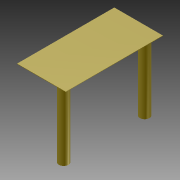
# Autodesk Inventor part: A11P-toggle-terminals
Saved by Autodesk Inventor 2011 SP1 (Build 150282100, 282)
## iProperties
Created: 2013-12-24
Part Number: A11P-toggle-terminals
Catalog Web Link: www.cadenas.de
Description: A Series - Process Sealed Subminiature Toggle - terminals-
Vendor: NKKSWITCHES
Document SubType Name: Modeling
Designer: PARTuser1
Manufacturer: NKKSWITCHES
Density: 1 g/cm^3
Category: PARTsolutions
Company: NKKSWITCHES
Title: A11P-toggle-terminals
Author: Cadenas PARTsolutions
PSOL_IDENT_0: {$CADENAS_DATA\23d-libs\nkkswitches\toggle\a\parts\a_toggle_terminals.prj},251 {VTYP=3D},{NB=A11P-to
PSOL_IDENT_1: ggle-terminals},{LINA=A11P-toggle-terminals},{NN=A Series - Process Sealed Subminiature Toggle - ter
PSOL_IDENT_2: minals},{DATE=05.03.2009 11:13:08},{GEOMDATE=05.03.2009 00:00:00},{VERSION=},{LINEID=10},{LINESUBID=
PSOL_IDENT_3: -1},{WBVAR=PLS,TRMNLS,CRCTS}  {NB=A11P-toggle-terminals},{LINA=A11P-toggle-terminals},{KT=DUMMY},{PN
PSOL_IDENT_4: =A11P},{SRS=A},{PLS=1},{TRMNLS=P},{TRMNLS1= 'P', 'P - Straight', 'B', 'B - Straight with Bracket', '
PSOL_IDENT_5: B1', 'B1 - Straight with Inline Bracket', 'H', 'H - Right Angle with Bracket', 'V', 'V - Vertical wi
PSOL_IDENT_6: th Bracket', 'V1', 'V1 - Vertical with Inline Bracket', 'W', 'W - Straight Long' },{CRCTS=1},{CRCTS1
PSOL_IDENT_7: = '1', '1 - OFF/NONE/ON',  '2', '2 - ON/NONE/ON', '3', '3 - ON/OFF/ON', '5'  , '5 - ON/NONE/(ON)', '
PSOL_IDENT_8: R', 'R - (ON)/NONE/ON', '8', '8 - (ON)/OFF/(ON)', '9'  , '9 - ON/OFF/(ON)', 'S', 'S - (ON)/OFF/ON' }
CNS_NN: A Series - Process Sealed Subminiature Toggle - terminals
CNS_NB: A11P-toggle-terminals
CNS_NBSYN: $PN.-toggle-terminals
CNS_LINA: A11P-toggle-terminals
CNS_PN: A11P
CNS_SRS: A
CNS_PLS: 1 - SPST/SPDT
CNS_TRMNLS: P - Straight
CNS_TRMNLS1: 'P', 'P - Straight', 'B', 'B - Straight with Bracket', 'B1', 'B1 - Straight with Inline Bracket', 'H', 'H - Right Angle with Bracket', 'V', 'V - Vertical with Bracket', 'V1', 'V1 - Vertical with Inline Bracket', 'W', 'W - Straight Long'
CNS_CRCTS: 1 - OFF/NONE/ON
CNS_CRCTS1: '1', '1 - OFF/NONE/ON',  '2', '2 - ON/NONE/ON', '3', '3 - ON/OFF/ON', '5'  , '5 - ON/NONE/(ON)', 'R', 'R - (ON)/NONE/ON', '8', '8 - (ON)/OFF/(ON)', '9'  , '9 - ON/OFF/(ON)', 'S', 'S - (ON)/OFF/ON'
SUPPLIER: NKKSWITCHES
ARTICLENO: A11P-toggle-terminals
BOMINFO: A11P-toggle-terminals
CREATOR: CADENAS GmbH
Autodesk Inventor part; units mm, degrees
sketch "Sketch_1" plane through (0, 0, 0) normal (0, 1, 0) x (-1, 0, 0)
  line L0 (1.4224, 3.048) -> (-1.6256, 3.048)
  line L1 (-1.6256, 3.048) -> (-1.6256, -3.048)
  line L2 (-1.6256, -3.048) -> (1.4224, -3.048)
  line L3 (1.4224, -3.048) -> (1.4224, 3.048)
  constraints: 8 end point
extrude "Extrusion1" add sketch "Sketch_1" along normal blind 0.0254
sketch "Sketch_2" plane through (0, 0, 0) normal (0, 1, 0) x (-1, 0, 0)
  circle A0 centre (-0.9906, -2.54) radius 0.3048
  constraints: 1 centre point
extrude "Extrusion2" add sketch "Sketch_2" against normal blind 4.3688
pattern_linear "Rectangular Pattern1" count 2 spacing 5.08 along (0, 0, 1) of "Extrusion2"
ref_plane "to_body_XY" through (0, 0, 0) normal (0, -1, 0) x (1, 0, 0)
ref_plane "to_body_YZ" through (0, 0, 0) normal (1, 0, 0) x (0, 0, 1)
ref_plane "to_body_ZX" through (0, 0, 0) normal (0, 0, 1) x (0, -1, 0)
ref_plane "to_body1_XY" through (0, -0.1016, 0.0254) normal (0, -1, 0) x (1, 0, 0)
ref_plane "to_body1_YZ" through (0, -0.1016, 0.0254) normal (1, 0, 0) x (0, 0, 1)
ref_plane "to_body1_ZX" through (0, -0.1016, 0.0254) normal (0, 0, 1) x (0, -1, 0)
body "Solid1"
